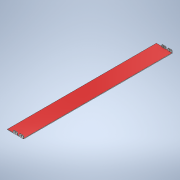
# Autodesk Inventor part: Caja - Pared
Saved by Autodesk Inventor 2021 (Build 250183000, 183)
## iProperties
Created: 2022-01-23
Part Number: Caja - Pared
Material: Generic
Document SubType Name: Modeling
Designer: deuts
Density: 1 g/cm^3
Appearance: Default
Author: deuts
Autodesk Inventor part; units mm, degrees
ref_plane "XZ Plane" through (0, 0, 0) normal (0, 1, 0) x (-1, 0, 0)
ref_plane "XY Plane" through (0, 0, 0) normal (0, 0, 1) x (1, 0, 0)
sketch "Sketch1" plane through (0, 0, 0) normal (0, 1, 0) x (-1, 0, 0)
  line L0 (24, 221.2) -> (24, -221.2)
  line L1 (-24, -220.2) -> (-24, 220.2)
  arc A0 (-23, 221.2) -> (-24, 220.2) centre (-23, 220.2) ccw
  arc A1 (-24, -220.2) -> (-23, -221.2) centre (-23, -220.2) ccw
  line L2 (0, 0) -> (-12.5, 0)
  line L3 (-23, 221.2) -> (24, 221.2)
  line L4 (-23, -221.2) -> (24, -221.2)
  point P0 (-24, -221.2)
  dimension "d0" = 442.4
  dimension "d1" = 48
  dimension "d2" = 1
  dimension "d3" = 1
  dimension "d58" = 221.2
  constraints: 10 end point, 4 point on circle, 3 horizontal, 2 centre point, 2 tangent, 1 parallel, 1 point on line
  measures "d0" distance of L0.start L0.end
  measures "d1" distance of L0.end point (-24, -221.2)
  measures "d2" radius of A0
  measures "d3" radius of A1
  measures "d58" distance from line of L4 L2.start
extrude "Extrusion1" add sketch "Sketch1" along normal blind 1.6
ref_plane "Work Plane1" through (7.995, 0, 0) normal (1, 0, 0) x (0, 1, 0)
sketch "Sketch4" plane through (0, 1.6, 0) normal (0, 1, 0) x (1, 0, 0)
  line L0 (-24, -221.2) -> (23, -221.2) projected
  line L1 (23, -221.2) -> (15, -221.2)
  line L2 (11, -219.6) -> (23, -219.6)
  line L3 (23, -219.6) -> (23, -221.2)
  line L4 (23, -221.2) -> (11, -221.2)
  line L5 (11, -221.2) -> (11, -219.6)
  line L6 (23, -221.2) -> (22, -221.2)
  line L7 (24, -220.2) -> (24, 220.2) projected
  point P0 (0, 0)
  dimension "d46" = 8
  dimension "d48" = 12
  dimension "d57" = 1
  constraints: 12 end point, 2 parallel, 2 point on line, 1 horizontal, 1 perpendicular
  measures "d46" distance of L0.end L1.end
  measures "d48" distance of L3.end L4.end
  measures "d57" distance between parallel lines of L7 L3
extrude "Extrusion4" add sketch "Sketch4" along normal blind 6
sketch "Sketch5" plane through (-24, 0, 221.2) normal (0, 0, 1) x (1, 0, 0)
  line L0 (35, 1.6) -> (47, 1.6) projected
  line L1 (47, 1.6) -> (47, 7.6) projected
  line L2 (47, 7.6) -> (35, 7.6) projected
  line L3 (0, 1.6) -> (35, 1.6) projected
  circle A0 centre (40.9972, 4.6) radius 2
  line L4 (35, 1.6) -> (47, 7.6)
  line L5 (35, 7.6) -> (47, 1.6)
  point P0 (24, 0)
  dimension "d52" = 4
  constraints: 4 end point, 1 centre point
  measures "d52" diameter of A0
extrude "Extrusion5" cut sketch "Sketch5" against normal blind 6 contours L4 L5 A0 | A0 L5 L4 | L5 L4 A0 | A0 L4 L5
fillet "Fillet3" radius 2 2 edges at (23, 7.6, 220.4) (11, 7.6, 220.4)
mirror "Mirror5" about plane through (7.995, 0, 0) normal (1, 0, 0) of "Extrusion4", "Extrusion5", "Fillet3"
mirror "Mirror6" about plane through (0, 0, 0) normal (0, 0, 1) of "Extrusion4", "Extrusion5", "Fillet3", "Mirror5"
body "Solid1"
